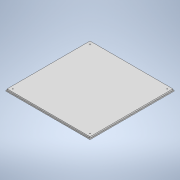
# Autodesk Inventor part: tapa_cuboLed
Saved by Autodesk Inventor 2021 (Build 250183000, 183)
## iProperties
Created: 2022-06-13
Part Number: tapa_cuboLed
Material: Genérico
Document SubType Name: Modeling
Designer: Dell
Density: 1 g/cm^3
Appearance: Valor por defecto
Author: Dell
Autodesk Inventor part; units mm, degrees
ref_plane "YZ Plane" through (0, 0, 0) normal (1, 0, 0) x (0, 1, 0)
ref_plane "XZ Plane" through (0, 0, 0) normal (0, 1, 0) x (-1, 0, 0)
ref_plane "XY Plane" through (0, 0, 0) normal (0, 0, 1) x (1, 0, 0)
sketch "Boceto1" plane through (0, 0, 0) normal (0, 1, 0) x (-1, 0, 0)
  line L0 (-103, 103) -> (103, 103)
  line L1 (103, 103) -> (103, -103)
  line L2 (103, -103) -> (-103, -103)
  line L3 (-103, -103) -> (-103, 103)
  line L4 (-103, 103) -> (103, -103) construction
  line L5 (103, 103) -> (-103, -103) construction
  point P0 (0, 0)
  dimension "d0" = 206
  dimension "d1" = 206
  constraints: 12 end point, 2 midpoint, 2 parallel, 1 horizontal, 1 perpendicular
  measures "d0" distance of L1.end L2.end
  measures "d1" distance of L0.end L1.end
extrude "Extrusión1" add sketch "Boceto1" along normal blind 5
sketch "Boceto3" plane through (0, 5, 0) normal (0, 1, 0) x (1, 0, 0)
  line L0 (85, 100) -> (103, 100)
  line L1 (103, -103) -> (103, 103) projected
  line L2 (100, -85) -> (100, 85) projected
  line L3 (100, 85) -> (100, 100)
  line L4 (100, 100) -> (116.202, 100) construction
  arc A0 (85, 100) -> (100, 85) centre (100, 100) ccw projected
  line L5 (89.3934, 89.3934) -> (89.3934, 100)
  line L6 (89.3934, 89.3934) -> (100, 89.3934)
  line L7 (89.3934, 100) -> (100, 89.3934)
  line L8 (89.3934, 89.3934) -> (100, 100)
  circle A1 centre (94.6967, 94.6967) radius 1
  circle A2 centre (-94.6967, 94.6967) radius 1
  circle A3 centre (-94.6967, -94.6967) radius 1
  circle A4 centre (94.6967, -94.6967) radius 1
  point P0 (0, 0)
  dimension "d12" = 2
  dimension "d15" = 360
  constraints: 14 end point, 4 centre point, 4 perpendicular, 4 point on line, 2 horizontal, 1 midpoint, 1 point on circle, 9 other
  measures "d12" diameter of A1
hole "Agujero1" at (-94.6967, 5, -94.6967) at (-94.6967, 5, 94.6967) at (94.6967, 5, 94.6967) at (94.6967, 5, -94.6967) direction (0, -1, 0) diameter 2 end through all
sketch "Boceto4" plane through (0, 5, 0) normal (0, 1, 0) x (1, 0, 0)
  line L0 (-101.5, 101.5) -> (101.5, 101.5)
  line L1 (101.5, 101.5) -> (101.5, -101.5)
  line L2 (101.5, -101.5) -> (-101.5, -101.5)
  line L3 (-101.5, -101.5) -> (-101.5, 101.5)
  line L4 (-101.5, 101.5) -> (101.5, -101.5) construction
  line L5 (101.5, 101.5) -> (-101.5, -101.5) construction
  line L6 (-103, -103) -> (103, -103)
  line L7 (103, -103) -> (103, 103)
  line L8 (103, 103) -> (-103, 103)
  line L9 (-103, 103) -> (-103, -103)
  point P0 (0, 0)
  dimension "d24" = 203
  dimension "d25" = 203
  dimension "d26" = 206
  dimension "d27" = 206
  constraints: 20 end point, 4 parallel, 2 horizontal, 2 midpoint, 2 perpendicular
  measures "d24" distance of L1.end L2.end
  measures "d25" distance of L0.end L1.end
  measures "d26" distance of L8.end L7.end
  measures "d27" distance of L7.end L6.end
extrude "Extrusión3" cut sketch "Boceto4" against normal blind 3
sketch "Boceto5" plane through (0, 0, 0) normal (0, -1, 0) x (1, 0, 0)
  point P0 (0, 0)
sketch "Boceto6" plane through (0, 0, 0) normal (0, -1, 0) x (1, 0, 0)
  point P0 (0, 0)
